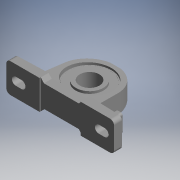
# Autodesk Inventor part: PDRM50_b
Saved by Autodesk Inventor 2017.3 (Build 213256000, 256)
## iProperties
Part Number: PDRM50_b
Material: Generic
Catalog Web Link: www.cadenas.de
Description: PDRM_body-Ball Bearing Units - Pillow Casting Housing Type -
Vendor: MISUMI
Document SubType Name: Modeling
Designer: partserver
Manufacturer: MISUMI
Mass: 930.047 g
Surface Area: 1139.51 cm^2
Volume: 930.047 cm^3
Density: 1 g/cm^3
Appearance: PSOLRGB-175-175-175
Category: PARTsolutions
Company: MISUMI
Title: PDRM50
Author: Cadenas PARTsolutions
Comments: Ball Bearing Units - Pillow Casting Housing Type -
PSOL_IDENT_0: {$CADENAS_DATA\23d-libs\misumi\metric\12_bearing_holders\pdrm\pdrm_body.prj},157 {VTYP=3D},{NB=PDRM5
PSOL_IDENT_1: 0_b},{LINA=PDRM50},{NN=PDRM_body},{DATE=18.09.2019 02:28:40},{GEOMDATE=03.09.2019 08:48:32},{VERSION=
PSOL_IDENT_2: },{LINEID=60},{WBVAR=},{WBNUMERIC=}  {NB=PDRM50_b},{LINA=PDRM50},{KT=DUMMY},{PN=PDRM50},{TYPE=PDRM},
PSOL_IDENT_3: {MTH=Alloy Cast Iron Class No.30},{MTB=52100 Bearing Steel},{MTRS=Silicon Rubber},{MTSS=4137 Alloy S
PSOL_IDENT_4: teel},{PRECISION=JIS B 1558, JIS B 1559},{OT=-15 ~+100},{D=50},{JIS=UCP310},{H=75},{L=275},{L1=212},
PSOL_IDENT_5: {A=75},{DD1=35},{DD=20},{TT=28},{H1=143},{B=61},{S=22},{CRR=61.5},{COR=38.2},{M1=M12x1.5},{M1ALG=12}
PSOL_IDENT_6: ,{T=2790},{ALC=3075},{MASS=5680},{HR1=68},{HR2=111},{HR3=105.243},{HR4=70.5},{HH1=20},{HH2=23},{HW2=
PSOL_IDENT_7: 89},{HW3=105},{HW4=143.0},{HA1=3.695},{HW5=56.5},{HW6=40},{R1=5},{R2=18},{R3=10},{LEN1=131.5},{LEN2=
PSOL_IDENT_8: 18},{W=36},{BW=32},{GZ=9.0},{LS=12}
NB: PDRM50_b
NN: PDRM_body
NT: Ball Bearing Units - Pillow Casting Housing Type -
NBSYN: $PN._b
LINA: PDRM50
CATALOG: Misumi
PN: PDRM50
TYPE: PDRM
MTH: Alloy Cast Iron Class No.30
MTB: 52100 Bearing Steel
MTRS: Silicon Rubber
MTSS: 4137 Alloy Steel
PRECISION: JIS B 1558, JIS B 1559
OT: -15 ~+100
D: 50
JIS: UCP310
H: 75
L: 275
L1: 212
A: 75
DD1: 35
DD: 20
TT: 28
H1: 143
B: 61
S: 22
CRR: 61.5
COR: 38.2
M1: M12x1.5
T: 2790
ALC: 3075
MASS: 5680
SUPPLIER: MISUMI
ARTICLENO: PDRM50_b
BOMINFO: PDRM50
CREATOR: CADENAS GmbH
Autodesk Inventor part; units mm, degrees
sketch "_____1" plane through (0, 0, 0) normal (0, 0, 1) x (1, 0, 0)
  line L0 (-71.5, -52) -> (71.5, -52)
  line L1 (71.5, -52) -> (67.8589, 4.3821)
  arc A0 (67.8589, 4.3821) -> (-67.8589, 4.3821) centre (0, -0.0002) ccw
  line L2 (-67.8589, 4.3821) -> (-71.5, -52)
  constraints: 6 end point, 2 point on circle, 1 centre point
extrude "Extrusion1" add sketch "_____1" along normal mid plane 75
sketch "_____2" plane through (0, 0, 0) normal (1, 0, 0) x (0, 1, 0)
  line L0 (71, 37.5) -> (-52, 37.5)
  line L1 (-52, 37.5) -> (-52, 28.25)
  line L2 (-52, 28.25) -> (66.5945, 20)
  arc A0 (66.5945, -20) -> (66.5945, 20) centre (-75, 0) ccw
  line L3 (66.5945, -20) -> (-52, -28.25)
  line L4 (-52, -28.25) -> (-52, -37.5)
  line L5 (-52, -37.5) -> (71, -37.5)
  line L6 (71, -37.5) -> (71, 37.5)
  constraints: 14 end point, 2 point on circle, 1 centre point
extrude "Extrusion2" cut sketch "_____2" along normal mid plane 150
sketch "_____3" plane through (0, 0, 0) normal (0, 0, 1) x (1, 0, 0)
  line L0 (-137.5, -55) -> (-137.5, -75)
  line L1 (-137.5, -75) -> (137.5, -75)
  line L2 (137.5, -75) -> (137.5, -55)
  line L3 (137.5, -55) -> (44.5, -52)
  line L4 (44.5, -52) -> (-44.5, -52)
  line L5 (-44.5, -52) -> (-137.5, -55)
  constraints: 12 end point
extrude "Extrusion3" add sketch "_____3" along normal mid plane 75
sketch "_____4" plane through (0, -47, 0) normal (0, 1, 0) x (1, 0, 0)
  line L0 (0, -18) -> (108.5, -18)
  arc A0 (113.5, -23) -> (108.5, -18) centre (108.5, -23) ccw
  line L1 (113.5, -23) -> (113.5, -32.5)
  arc A1 (113.5, -32.5) -> (118.5, -37.5) centre (118.5, -32.5) ccw
  line L2 (118.5, -37.5) -> (126.5, -37.5)
  arc A2 (126.5, -37.5) -> (131.5, -32.5) centre (126.5, -32.5) ccw
  line L3 (131.5, -32.5) -> (131.5, 0)
  arc A3 (131.5, 0) -> (113.5, 18) centre (113.5, 0) ccw
  line L4 (113.5, 18) -> (0, 18)
  line L5 (0, 18) -> (0, -18)
  constraints: 12 end point, 8 point on circle, 4 centre point
extrude "Extrusion4" add sketch "_____4" against normal blind 28
sketch "_____5" plane through (0, -47, 0) normal (0, 1, 0) x (1, 0, 0)
  line L0 (-131.5, 32.5) -> (-131.5, 0)
  arc A0 (-131.5, 0) -> (-113.5, -18) centre (-113.5, 0) ccw
  line L1 (-113.5, -18) -> (0, -18)
  line L2 (0, -18) -> (0, 18)
  line L3 (0, 18) -> (-108.5, 18)
  arc A1 (-113.5, 23) -> (-108.5, 18) centre (-108.5, 23) ccw
  line L4 (-113.5, 23) -> (-113.5, 32.5)
  arc A2 (-113.5, 32.5) -> (-118.5, 37.5) centre (-118.5, 32.5) ccw
  line L5 (-118.5, 37.5) -> (-126.5, 37.5)
  arc A3 (-126.5, 37.5) -> (-131.5, 32.5) centre (-126.5, 32.5) ccw
  constraints: 12 end point, 8 point on circle, 4 centre point
extrude "Extrusion5" add sketch "_____5" against normal blind 28
sketch "_____6" plane through (0, -47, 0) normal (0, 1, 0) x (1, 0, 0)
  line L0 (-140.5, 40.5) -> (-140.5, -40.5)
  line L1 (-140.5, -40.5) -> (140.5, -40.5)
  line L2 (140.5, -40.5) -> (140.5, 40.5)
  line L3 (140.5, 40.5) -> (-140.5, 40.5)
  line L4 (-137.5, 27.5) -> (-137.5, -27.5)
  arc A0 (-137.5, -27.5) -> (-127.5, -37.5) centre (-127.5, -27.5) ccw
  line L5 (-127.5, -37.5) -> (-52.5, -37.5)
  line L6 (-52.5, -37.5) -> (-44.5, -28.25)
  line L7 (-44.5, -28.25) -> (44.5, -28.25)
  line L8 (44.5, -28.25) -> (52.5, -37.5)
  line L9 (52.5, -37.5) -> (127.5, -37.5)
  arc A1 (127.5, -37.5) -> (137.5, -27.5) centre (127.5, -27.5) ccw
  line L10 (137.5, -27.5) -> (137.5, 27.5)
  arc A2 (137.5, 27.5) -> (127.5, 37.5) centre (127.5, 27.5) ccw
  line L11 (127.5, 37.5) -> (52.5, 37.5)
  line L12 (52.5, 37.5) -> (44.5, 28.25)
  line L13 (44.5, 28.25) -> (-44.5, 28.25)
  line L14 (-44.5, 28.25) -> (-52.5, 37.5)
  line L15 (-52.5, 37.5) -> (-127.5, 37.5)
  arc A3 (-127.5, 37.5) -> (-137.5, 27.5) centre (-127.5, 27.5) ccw
  constraints: 32 end point, 8 point on circle, 4 centre point
extrude "Extrusion6" cut sketch "_____6" against normal blind 28
sketch "_____7" plane through (0, -47, 0) normal (0, 1, 0) x (1, 0, 0)
  arc A0 (98.5, 10) -> (98.5, -10) centre (98.5, 0) ccw
  line L0 (98.5, -10) -> (113.5, -10)
  arc A1 (113.5, -10) -> (113.5, 10) centre (113.5, 0) ccw
  line L1 (113.5, 10) -> (98.5, 10)
  constraints: 4 end point, 4 point on circle, 2 centre point
extrude "Extrusion7" cut sketch "_____7" against normal blind 28
sketch "_____8" plane through (0, -47, 0) normal (0, 1, 0) x (1, 0, 0)
  arc A0 (-113.5, 10) -> (-113.5, -10) centre (-113.5, 0) ccw
  line L0 (-113.5, -10) -> (-98.5, -10)
  arc A1 (-98.5, -10) -> (-98.5, 10) centre (-98.5, 0) ccw
  line L1 (-98.5, 10) -> (-113.5, 10)
  constraints: 4 end point, 4 point on circle, 2 centre point
extrude "Extrusion8" cut sketch "_____8" against normal blind 28
sketch "_____9" plane through (0, 0, 0) normal (1, 0, 0) x (0, 1, 0)
  line L0 (0, -32) -> (0, -16)
  line L1 (0, -16) -> (55.5, -16)
  line L2 (55.5, -16) -> (55.5, -32)
  line L3 (55.5, -32) -> (0, -32)
  line L4 (0, -32) -> (0, -16)
  constraints: 10 end point
revolve "Revolution1" cut sketch "_____9" angle 360 about axis through (0, 0, -32) along (0, 0, -1)
sketch "_____10" plane through (0, 0, 0) normal (1, 0, 0) x (0, 1, 0)
  line L0 (0, 16) -> (0, 32)
  line L1 (0, 32) -> (55.5, 32)
  line L2 (55.5, 32) -> (55.5, 16)
  line L3 (55.5, 16) -> (0, 16)
  line L4 (0, 16) -> (0, 32)
  constraints: 10 end point
revolve "Revolution2" cut sketch "_____10" angle 360 about axis through (0, 0, 16) along (0, 0, -1)
sketch "_____11" plane through (0, 0, 0) normal (1, 0, 0) x (0, 1, 0)
  line L0 (0, -50) -> (0, 50)
  arc A0 (52.6715, -16) -> (52.5715, -16) centre (52.6215, -16) ccw
  line L1 (52.5715, -16) -> (52.6715, -16)
  constraints: 4 end point, 2 point on circle, 1 centre point
revolve "Revolution3" cut sketch "_____11" angle 360 about axis through (0, 0, -50) along (0, 0, -1)
sketch "_____12" plane through (0, 0, 0) normal (1, 0, 0) x (0, 1, 0)
  line L0 (0, -50) -> (0, 50)
  line L1 (52.6715, 16) -> (52.5715, 16)
  arc A0 (52.5715, 16) -> (52.6715, 16) centre (52.6215, 16) ccw
  constraints: 4 end point, 2 point on circle, 1 centre point
revolve "Revolution4" cut sketch "_____12" angle 360 about axis through (0, 0, -50) along (0, 0, -1)
sketch "_____13" plane through (0, 0, 0) normal (1, 0, 0) x (0, 1, 0)
  line L0 (0, -22) -> (0, 39)
  line L1 (0, 39) -> (35.25, 39)
  line L2 (35.25, 39) -> (35.25, -22)
  line L3 (35.25, -22) -> (0, -22)
  line L4 (0, -22) -> (0, 39)
  constraints: 10 end point
revolve "Revolution5" add sketch "_____13" angle 360 about axis through (0, 0, -22) along (0, 0, -1)
sketch "Sketch14" plane through (0, 0, -22) normal (0, 0, -1) x (-1, 0, 0)
  point P0 (0, 0)
hole "Hole1" at (0, 0, -22) direction (0, 0, 1) diameter 50 depth 61
sketch "_____15" plane through (0, 0, 0) normal (1, 0, 0) x (0, 1, 0)
  line L0 (24.5, 27) -> (35.25, 27)
  line L1 (35.25, 27) -> (35.25, 21)
  line L2 (35.25, 21) -> (34.303, 21.947)
  line L3 (34.303, 21.947) -> (24.5, 21.947)
  line L4 (24.5, 21.947) -> (24.5, 27)
  line L5 (24.5, 27) -> (35.25, 27)
  constraints: 12 end point
revolve "Revolution6" cut sketch "_____15" angle 360 about axis through (0, 24.5, 27) along (0, -1, 0)
thread "Thread1" size "M12x1.75" class "6H" standard "ISO Metric profile" full length
sketch "_____16" plane through (0, 0, 0) normal (-0.5, 0.8660254, 0) x (0, 0, -1)
  line L0 (-27, 24.5) -> (-27, 35.25)
  line L1 (-27, 35.25) -> (-21, 35.25)
  line L2 (-21, 35.25) -> (-21.947, 34.303)
  line L3 (-21.947, 34.303) -> (-21.947, 24.5)
  line L4 (-21.947, 24.5) -> (-27, 24.5)
  line L5 (-27, 24.5) -> (-27, 35.25)
  constraints: 12 end point
revolve "Revolution7" cut sketch "_____16" angle 360 about axis through (-21.2176, -12.25, 27) along (0.8660254, 0.5, 0)
thread "Thread2" size "M12x1.75" class "6H" standard "ISO Metric profile" full length
sketch "_____19" plane through (0, 0, 9) normal (0, 0, 1) x (1, 0, 0)
  line L0 (0, 77.1) -> (0, 67.25)
  line L1 (0, 67.25) -> (-3.3, 67.25)
  line L2 (-3.3, 67.25) -> (-3.3, 68.5)
  line L3 (-3.3, 68.5) -> (-3.5, 68.5)
  line L4 (-3.5, 68.5) -> (-5.2321, 69.5)
  line L5 (-5.2321, 69.5) -> (-3.5, 70.5)
  arc A0 (-3.5, 70.5) -> (-2.853, 72.2508) centre (-8.736, 73.4299) ccw
  arc A1 (-2.853, 72.2508) -> (-2.9276, 72.7772) centre (-3.6374, 72.4081) ccw
  arc A2 (-3.3, 74.3) -> (-2.9276, 72.7772) centre (0, 74.3) ccw
  line L6 (-3.3, 74.3) -> (-2.4, 77)
  line L7 (-2.4, 77) -> (-0.5546, 77)
  arc A3 (0, 77.1) -> (-0.5546, 77) centre (0, 75.512) ccw
  line L8 (0, 77.1) -> (0, 67.25)
  constraints: 18 end point, 8 point on circle, 4 centre point
revolve "Revolution8" add sketch "_____19" angle 360 about axis through (0, 77.1, 9) along (0, 1, 0)
sketch "_____20" plane through (0, 68, 0) normal (0, 1, 0) x (1, 0, 0)
  circle A0 centre (0, -9) radius 10
  line L0 (-4.0415, -9) -> (-2.0207, -12.5)
  line L1 (-2.0207, -12.5) -> (2.0207, -12.5)
  line L2 (2.0207, -12.5) -> (4.0415, -9)
  line L3 (4.0415, -9) -> (2.0207, -5.5)
  line L4 (2.0207, -5.5) -> (-2.0207, -5.5)
  line L5 (-2.0207, -5.5) -> (-4.0415, -9)
  constraints: 12 end point, 1 centre point
extrude "Extrusion9" cut sketch "_____20" along normal blind 4
sketch "_____21" plane through (0, 0, 0) normal (0, 0, 1) x (1, 0, 0)
  line L0 (-52.5, -72) -> (-52.5, -75)
  line L1 (-52.5, -75) -> (52.5, -75)
  line L2 (52.5, -75) -> (52.5, -72)
  line L3 (52.5, -72) -> (-52.5, -72)
  constraints: 8 end point
extrude "Extrusion10" cut sketch "_____21" along normal mid plane 150
ref_plane "cp1_XY" through (0, 25, 27) normal (0, 1, 0) x (1, 0, 0)
ref_plane "cp1_YZ" through (0, 25, 27) normal (1, 0, 0) x (0, 0, -1)
ref_plane "cp1_ZX" through (0, 25, 27) normal (0, 0, -1) x (0, 1, 0)
ref_plane "cp2_XY" through (-21.6506, -12.5, 27) normal (-0.8660254, -0.5, 0) x (-0.5, 0.8660254, 0)
ref_plane "cp2_YZ" through (-21.6506, -12.5, 27) normal (-0.5, 0.8660254, 0) x (0, 0, -1)
ref_plane "cp2_ZX" through (-21.6506, -12.5, 27) normal (0, 0, -1) x (-0.8660254, -0.5, 0)
body "Solid1"
